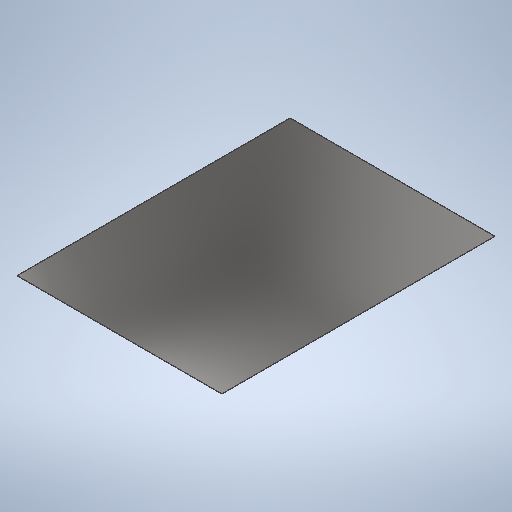
# Autodesk Inventor part: field_plate_SUS4301
Saved by Autodesk Inventor 2025 (Build 290162000, 162)
## iProperties
Created: 2026-02-16
Part Number: field_plate_SUS4301
Material: 一般
Document SubType Name: Modeling
Designer: sooo1
Density: 1 g/cm^3
Appearance: 鋼 - つや出し
Author: sooo1
Autodesk Inventor part; units mm, degrees
ref_plane "YZ Plane" through (0, 0, 0) normal (1, 0, 0) x (0, 1, 0)
ref_plane "XZ Plane" through (0, 0, 0) normal (0, 1, 0) x (-1, 0, 0)
ref_plane "XY Plane" through (0, 0, 0) normal (0, 0, 1) x (1, 0, 0)
sketch "スケッチ1" plane through (0, 0, 0) normal (0, 1, 0) x (-1, 0, 0)
  line L0 (150, 200) -> (-150, 200)
  line L1 (-150, 200) -> (-150, -200)
  line L2 (-150, -200) -> (150, -200)
  line L3 (150, -200) -> (150, 200)
  line L4 (150, 200) -> (-150, -200) construction
  line L5 (-150, 200) -> (150, -200) construction
  point P0 (0, 0)
  dimension "d0" = 400
  dimension "d1" = 300
  constraints: 12 end point, 2 midpoint, 2 parallel, 1 horizontal, 1 perpendicular
  measures "d0" distance of L2.end L0.start
  measures "d1" distance of L0.start L0.end
extrude "押し出し1" add sketch "スケッチ1" along normal blind 0.5
